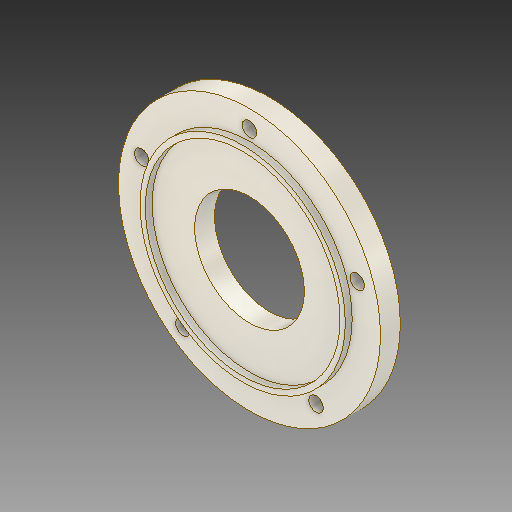
# Autodesk Inventor part: 301-03
Saved by Autodesk Inventor 2019 (Build 230136000, 136)
## iProperties
Company: Autodesk Inc.
Created: 2017-03-16
Part Number: 301-03
Material: Titanium
Document SubType Name: Modeling
Designer: Autodesk Inc.
Density: 4.51 g/cm^3
Appearance: Titanium
Mass: 89.252 g
Surface Area: 98.5071 cm^2
Volume: 19.7898 cm^3
Author: Inventor
Autodesk Inventor part; units mm, degrees
ref_plane "YZ Plane" through (0, 0, 0) normal (1, 0, 0) x (0, 1, 0)
ref_plane "XZ Plane" through (0, 0, 0) normal (0, 1, 0) x (-1, 0, 0)
ref_plane "XY Plane" through (0, 0, 0) normal (0, 0, 1) x (1, 0, 0)
sketch "Sketch1" plane through (0, 0, 0) normal (0, 0, 1) x (1, 0, 0)
  circle A0 centre (0, 0) radius 15.5
  circle A1 centre (0, 0) radius 37
  dimension "d0" = 31
  dimension "d1" = 74
  constraints: 2 centre point, 2 coincident
  measures "d0" diameter of A0
  measures "d1" diameter of A1
extrude "Extrusion1" add sketch "Sketch1" along normal mid plane 5.606
sketch "Sketch2" plane through (0, 0, 2.803) normal (0, 0, 1) x (1, 0, 0)
  circle A0 centre (0, 0) radius 37 projected
  circle A1 centre (0, 0) radius 27.5
  circle A2 centre (0, 0) radius 29
  dimension "d4" = 55
  dimension "d5" = 58
  constraints: 2 centre point, 2 coincident
  measures "d4" diameter of A1
  measures "d5" diameter of A2
extrude "Extrusion2" add sketch "Sketch2" along normal blind 1.936 contours A2
ref_plane "Work Plane1" through (0, 0, -2.088) normal (0, 0, -1) x (-1, 0, 0)
sketch "Sketch3" plane through (0, 0, -2.088) normal (0, 0, -1) x (-1, 0, 0)
  circle A0 centre (0, 0) radius 15.5 projected
  point P0 (0, 32)
  dimension "d9" = 32
  constraints: 1 vertical alignment
  measures "d9" distance of A0.centre point (0, 32)
hole "Hole1" at (0, 32, -2.088) direction (0, 0, 1) diameter 4.117 end through all start extended yes countersink diameter 7.53 countersink angle 90
pattern_circular "Circular Pattern1" count 5 over 360 about axis through (0, 0, -10) along (0, 0, 1) of "Hole1"
body "Solid1"
